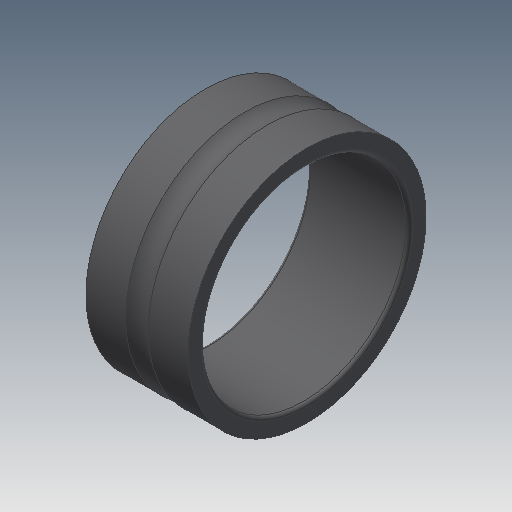
# Autodesk Inventor part: MF106ZZ1 Inner Ring
Saved by Autodesk Inventor 2019.4 (Build 234330000, 330)
## iProperties
Category: PARTsolutions
Company: NSK_RB
Created: 2019-11-13
Part Number: MF106ZZ1 Inner Ring
Material: 一般
Catalog Web Link: www.cadenas.de
Description: shielded_type_zz_zzs_IR-
Vendor: NSK_RB
Document SubType Name: Modeling
Designer: psadmin
Manufacturer: NSK_RB
Mass: 0.0295705 g
Surface Area: 1.41909 cm^2
Volume: 0.0295705 cm^3
Density: 1 g/cm^3
Appearance: PSOLRGB-128-128-128
PSOL_IDENT_0: {$CADENAS_DATA\23d-libs\nsk_rb\roller_bearings\deep_groove_bb\exstra_small_miniatur_bb\metric_design
PSOL_IDENT_1: _with_flange\shielded_type_zz_zzs_ir_1.prj},196 {VTYP=3D},{NB=MF106ZZ1 Inner Ring},{LINA=MF106ZZ1 In
PSOL_IDENT_2: ner Ring},{NN=shielded_type_zz_zzs_IR},{DATE=16.01.2019 01:41:16},{GEOMDATE=04.01.2008 00:00:00},{VE
PSOL_IDENT_3: RSION=},{LINEID=580},{WBVAR=},{WBNUMERIC=}  {NB=MF106ZZ1 Inner Ring},{LINA=MF106ZZ1 Inner Ring},{KT=
PSOL_IDENT_4: DUMMY},{IDNR=},{STAN=},{ORDER=MF106ZZ1},{SD=6.0},{X=6.0},{D=10},{DD=10},{DD1=0.0},{D2=11.2},{DD2=11.
PSOL_IDENT_5: 2},{B=0.0},{B1=3.0},{CC1=0.0},{C2=0.6},{CC2=0.6},{R=0.00},{R1=0.10},{DI1=7.00},{DI2=7.00},{SDE1=8.75
PSOL_IDENT_6: },{SDE2=9.31},{CR1=495},{COR1=218},{CR2=51},{COR2=22.0},{LG=45000},{LO=53000},{DA=0.0},{DB=7.0},{RA=
PSOL_IDENT_7: 0.00},{RB=0.10},{MASS=0.77},{SC=1},{N=16}
NN: shielded_type_zz_zzs_IR
NB: MF106ZZ1 Inner Ring
NBSYN: $ORDER. Inner Ring
LINA: MF106ZZ1 Inner Ring
ORDER: MF106ZZ1
SD: 6
X: 6
D: 10
DD: 10
DD1: 0
D2: 11.2
DD2: 11.2
B: 0
B1: 3
CC1: 0
C2: 0.6
CC2: 0.6
R: 0
R1: 0.1
DI1: 7
DI2: 7
SDE1: 8.75
SDE2: 9.31
CR1: 495
COR1: 218
CR2: 51
COR2: 22
LG: 45000
LO: 53000
DA: 0
DB: 7
RA: 0
RB: 0.1
MASS: 0.77
SC: 1
SUPPLIER: NSK_RB
ARTICLENO: MF106ZZ1 Inner Ring
BOMINFO: MF106ZZ1 Inner Ring
CREATOR: CADENAS GmbH
Title: MF106ZZ1 Inner Ring
Author: Cadenas PARTsolutions
Autodesk Inventor part; units mm, degrees
sketch "Sketch_1" plane through (0, 0, 0) normal (0, 0, 1) x (1, 0, 0)
  line L0 (3, 0) -> (0, 0)
  arc A0 (0, 3.1) -> (0.1, 3) centre (0.1, 3.1) ccw
  line L1 (0.1, 3) -> (2.9, 3)
  arc A1 (2.9, 3) -> (3, 3.1) centre (2.9, 3.1) ccw
  line L2 (3, 3.1) -> (3, 3.5)
  line L3 (3, 3.5) -> (1.8317, 3.5)
  arc A2 (1.1683, 3.5) -> (1.8317, 3.5) centre (1.5, 4) ccw
  line L4 (1.1683, 3.5) -> (0, 3.5)
  line L5 (0, 3.5) -> (0, 3.1)
  constraints: 12 end point, 6 point on circle, 3 centre point
revolve "Revolution1" add sketch "Sketch_1" angle 360 about axis through (3, 0, 0) along (1, 0, 0)
ref_plane "ip_st_1_1_XY" through (1.5, 4, 0) normal (1, 0, 0) x (0, 0, -1)
ref_plane "ip_st_1_1_YZ" through (1.5, 4, 0) normal (0, 0, -1) x (0, 1, 0)
ref_plane "ip_st_1_1_ZX" through (1.5, 4, 0) normal (0, 1, 0) x (1, 0, 0)
ref_plane "ip_st_1_10_XY" through (1.5, -3.6955, -1.5307) normal (1, 0, 0) x (0, 0, -1)
ref_plane "ip_st_1_10_YZ" through (1.5, -3.6955, -1.5307) normal (0, 0, -1) x (0, 1, 0)
ref_plane "ip_st_1_10_ZX" through (1.5, -3.6955, -1.5307) normal (0, 1, 0) x (1, 0, 0)
ref_plane "ip_st_1_11_XY" through (1.5, -2.8284, -2.8284) normal (1, 0, 0) x (0, 0, -1)
ref_plane "ip_st_1_11_YZ" through (1.5, -2.8284, -2.8284) normal (0, 0, -1) x (0, 1, 0)
ref_plane "ip_st_1_11_ZX" through (1.5, -2.8284, -2.8284) normal (0, 1, 0) x (1, 0, 0)
ref_plane "ip_st_1_12_XY" through (1.5, -1.5307, -3.6955) normal (1, 0, 0) x (0, 0, -1)
ref_plane "ip_st_1_12_YZ" through (1.5, -1.5307, -3.6955) normal (0, 0, -1) x (0, 1, 0)
ref_plane "ip_st_1_12_ZX" through (1.5, -1.5307, -3.6955) normal (0, 1, 0) x (1, 0, 0)
ref_plane "ip_st_1_13_XY" through (1.5, 0, -4) normal (1, 0, 0) x (0, 0, -1)
ref_plane "ip_st_1_13_YZ" through (1.5, 0, -4) normal (0, 0, -1) x (0, 1, 0)
ref_plane "ip_st_1_13_ZX" through (1.5, 0, -4) normal (0, 1, 0) x (1, 0, 0)
ref_plane "ip_st_1_14_XY" through (1.5, 1.5307, -3.6955) normal (1, 0, 0) x (0, 0, -1)
ref_plane "ip_st_1_14_YZ" through (1.5, 1.5307, -3.6955) normal (0, 0, -1) x (0, 1, 0)
ref_plane "ip_st_1_14_ZX" through (1.5, 1.5307, -3.6955) normal (0, 1, 0) x (1, 0, 0)
ref_plane "ip_st_1_15_XY" through (1.5, 2.8284, -2.8284) normal (1, 0, 0) x (0, 0, -1)
ref_plane "ip_st_1_15_YZ" through (1.5, 2.8284, -2.8284) normal (0, 0, -1) x (0, 1, 0)
ref_plane "ip_st_1_15_ZX" through (1.5, 2.8284, -2.8284) normal (0, 1, 0) x (1, 0, 0)
ref_plane "ip_st_1_16_XY" through (1.5, 3.6955, -1.5307) normal (1, 0, 0) x (0, 0, -1)
ref_plane "ip_st_1_16_YZ" through (1.5, 3.6955, -1.5307) normal (0, 0, -1) x (0, 1, 0)
ref_plane "ip_st_1_16_ZX" through (1.5, 3.6955, -1.5307) normal (0, 1, 0) x (1, 0, 0)
ref_plane "ip_st_1_2_XY" through (1.5, 3.6955, 1.5307) normal (1, 0, 0) x (0, 0, -1)
ref_plane "ip_st_1_2_YZ" through (1.5, 3.6955, 1.5307) normal (0, 0, -1) x (0, 1, 0)
ref_plane "ip_st_1_2_ZX" through (1.5, 3.6955, 1.5307) normal (0, 1, 0) x (1, 0, 0)
ref_plane "ip_st_1_3_XY" through (1.5, 2.8284, 2.8284) normal (1, 0, 0) x (0, 0, -1)
ref_plane "ip_st_1_3_YZ" through (1.5, 2.8284, 2.8284) normal (0, 0, -1) x (0, 1, 0)
ref_plane "ip_st_1_3_ZX" through (1.5, 2.8284, 2.8284) normal (0, 1, 0) x (1, 0, 0)
ref_plane "ip_st_1_4_XY" through (1.5, 1.5307, 3.6955) normal (1, 0, 0) x (0, 0, -1)
ref_plane "ip_st_1_4_YZ" through (1.5, 1.5307, 3.6955) normal (0, 0, -1) x (0, 1, 0)
ref_plane "ip_st_1_4_ZX" through (1.5, 1.5307, 3.6955) normal (0, 1, 0) x (1, 0, 0)
ref_plane "ip_st_1_5_XY" through (1.5, 0, 4) normal (1, 0, 0) x (0, 0, -1)
ref_plane "ip_st_1_5_YZ" through (1.5, 0, 4) normal (0, 0, -1) x (0, 1, 0)
ref_plane "ip_st_1_5_ZX" through (1.5, 0, 4) normal (0, 1, 0) x (1, 0, 0)
ref_plane "ip_st_1_6_XY" through (1.5, -1.5307, 3.6955) normal (1, 0, 0) x (0, 0, -1)
ref_plane "ip_st_1_6_YZ" through (1.5, -1.5307, 3.6955) normal (0, 0, -1) x (0, 1, 0)
ref_plane "ip_st_1_6_ZX" through (1.5, -1.5307, 3.6955) normal (0, 1, 0) x (1, 0, 0)
ref_plane "ip_st_1_7_XY" through (1.5, -2.8284, 2.8284) normal (1, 0, 0) x (0, 0, -1)
ref_plane "ip_st_1_7_YZ" through (1.5, -2.8284, 2.8284) normal (0, 0, -1) x (0, 1, 0)
ref_plane "ip_st_1_7_ZX" through (1.5, -2.8284, 2.8284) normal (0, 1, 0) x (1, 0, 0)
ref_plane "ip_st_1_8_XY" through (1.5, -3.6955, 1.5307) normal (1, 0, 0) x (0, 0, -1)
ref_plane "ip_st_1_8_YZ" through (1.5, -3.6955, 1.5307) normal (0, 0, -1) x (0, 1, 0)
ref_plane "ip_st_1_8_ZX" through (1.5, -3.6955, 1.5307) normal (0, 1, 0) x (1, 0, 0)
ref_plane "ip_st_1_9_XY" through (1.5, -4, 0) normal (1, 0, 0) x (0, 0, -1)
ref_plane "ip_st_1_9_YZ" through (1.5, -4, 0) normal (0, 0, -1) x (0, 1, 0)
ref_plane "ip_st_1_9_ZX" through (1.5, -4, 0) normal (0, 1, 0) x (1, 0, 0)
ref_plane "ip_st_1a_XY" through (0, 0, 0) normal (1, 0, 0) x (0, 0, -1)
ref_plane "ip_st_1a_YZ" through (0, 0, 0) normal (0, 0, -1) x (0, 1, 0)
ref_plane "ip_st_1a_ZX" through (0, 0, 0) normal (0, 1, 0) x (1, 0, 0)
ref_plane "ip_st_2a_XY" through (0.1875, 0, 0) normal (1, 0, 0) x (0, 0, -1)
ref_plane "ip_st_2a_YZ" through (0.1875, 0, 0) normal (0, 0, -1) x (0, 1, 0)
ref_plane "ip_st_2a_ZX" through (0.1875, 0, 0) normal (0, 1, 0) x (1, 0, 0)
body "Solid1"
